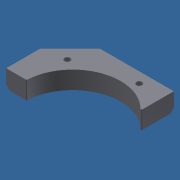
# Autodesk Inventor part: PÁRA-LAMAS DIANTEIRO-ESQ
Saved by Autodesk Inventor 2012 SP1 (Build 160190100, 190)
## iProperties
Created: 2012-07-24
Part Number: PÁRA-LAMAS DIANTEIRO-ESQ
Material: Carbon Steel
Document SubType Name: Modeling
Designer: bruno.silveira
Mass: 165.742 g
Surface Area: 61.02 cm^2
Volume: 21.06 cm^3
Density: 7.87 g/cm^3
Author: bruno.silveira
Autodesk Inventor part; units mm, degrees
ref_plane "YZ Plane" through (0, 0, 0) normal (1, 0, 0) x (0, 1, 0)
ref_plane "XZ Plane" through (0, 0, 0) normal (0, 1, 0) x (-1, 0, 0)
ref_plane "XY Plane" through (0, 0, 0) normal (0, 0, 1) x (1, 0, 0)
sketch "Sketch1" plane through (0, 0, 0) normal (0, 0, 1) x (1, 0, 0)
  line L0 (0, 0) -> (58.5, 0)
  line L1 (58.5, 0) -> (58.5, 36)
  line L2 (58.5, 36) -> (0, 36)
  line L3 (0, 36) -> (0, 0)
  dimension "d0" = 58.5
  dimension "d1" = 36
  constraints: 8 end point, 2 parallel, 1 horizontal, 1 perpendicular
  measures "d0" distance of L0.start L0.end
  measures "d1" distance of L2.end L0.start
extrude "Extrusion1" add sketch "Sketch1" along normal blind 10
sketch "Sketch2" plane through (0, 0, 10) normal (0, 0, 1) x (1, 0, 0)
  line L0 (0, 0) -> (0, 36) projected
  line L1 (58.5, 0) -> (0, 0) projected
  circle A0 centre (38.5, -1) radius 27
  dimension "d6" = 27
  dimension "d7" = 1
  dimension "d8" = 11.5
  constraints: 1 centre point
  measures "d6" radius of A0
  measures "d7" distance from line of L1 A0.centre
  measures "d8" distance edge to line of A0 L0
extrude "Extrusion2" cut sketch "Sketch2" against normal blind 10
sketch "Sketch3" plane through (0, 0, 10) normal (0, 0, 1) x (1, 0, 0)
  line L0 (58.5, 36) -> (58.5, 17.1384) projected
  line L1 (11.5185, 0) -> (0, 0) projected
  line L2 (0, 36) -> (58.5, 36) projected
  point P0 (13, 21.5)
  point P1 (45, 30)
  dimension "d11" = 32
  dimension "d12" = 13.5
  dimension "d13" = 21.5
  dimension "d28" = 6
  measures "d11" horizontal distance of point (45, 30) point (13, 21.5)
  measures "d12" distance from line of L0 point (45, 30)
  measures "d13" distance from line of L1 point (13, 21.5)
  measures "d28" distance from line of L2 point (45, 30)
hole "Hole1" at (13, 21.5, 10) at (45, 30, 10) direction (0, 0, -1) diameter 3.175 depth 10 tip angle 118
chamfer "Chamfer1" distance 17 angle 45 1 edges at (0, 36, 5)
chamfer "Chamfer2" distance 2 angle 45 3 edges at (37.75, 36, 0) (8.5, 27.5, 0) (0, 9.5, 0)
fillet "Fillet1" radius 0.5 2 edges at (58.5, 17.1384, 5) (11.5185, 0, 5)
body "Solid1"
